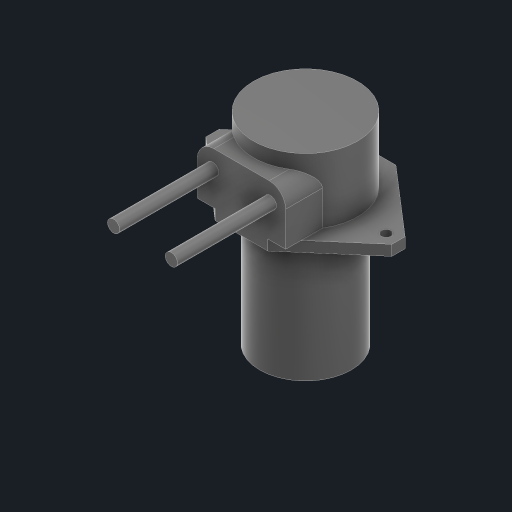
# Autodesk Inventor part: Peristaltic Pump
Saved by Autodesk Inventor 2023.1 (Build 271208000, 208)
## iProperties
Created: 2022-11-29
Part Number: Peristaltic Pump
Material: Acetal Resin, Black
Document SubType Name: Modeling
Designer: Jarrett
Density: 1.425 g/cm^3
Appearance: Smooth - Black
Author: Jarrett
Autodesk Inventor part; units mm, degrees
ref_plane "YZ Plane" through (0, 0, 0) normal (1, 0, 0) x (0, 1, 0)
ref_plane "XZ Plane" through (0, 0, 0) normal (0, 1, 0) x (-1, 0, 0)
ref_plane "XY Plane" through (0, 0, 0) normal (0, 0, 1) x (1, 0, 0)
sketch "Sketch1" plane through (0, 0, 0) normal (0, 1, 0) x (-1, 0, 0)
  line L0 (0, -19.39) -> (-8, -19.39)
  line L1 (-28.18, -2) -> (-28.18, 2)
  line L2 (-28.18, 2) -> (-8, 19.39)
  line L3 (-8, 19.39) -> (0, 19.39)
  circle A0 centre (-24.43, 0) radius 1.5
  circle A1 centre (0, 0) radius 15.75
  line L4 (0, -27.146) -> (0, 27.146) projected
  line L5 (-8, -19.39) -> (-28.18, -2)
  line L6 (39.452, 0) -> (-39.452, 0) projected
  line L7 (-13.385, 8.3009) -> (-13.385, 19.39)
  line L8 (-13.385, 19.39) -> (-8, 19.39)
  line L9 (0, -19.39) -> (8, -19.39)
  line L10 (28.18, -2) -> (28.18, 2)
  line L11 (28.18, 2) -> (8, 19.39)
  line L12 (8, 19.39) -> (0, 19.39)
  circle A2 centre (24.43, 0) radius 1.5
  line L13 (8, -19.39) -> (28.18, -2)
  line L14 (13.385, 8.3009) -> (13.385, 19.39)
  line L15 (13.385, 19.39) -> (8, 19.39)
  circle A3 centre (0, 0) radius 13.86
  point P0 (-28.18, 0)
  dimension "d4" = 31.5
  dimension "d0" = 56.36
  dimension "d1" = 38.78
  dimension "d2" = 4
  dimension "d3" = 16
  dimension "d5" = 26.77
  dimension "d6" = 3
  dimension "d7" = 3.75
  dimension "d8" = 27.72
  constraints: 28 end point, 7 symmetric about line, 3 centre point, 2 coincident, 2 perpendicular, 2 point on line, 1 equal length, 1 horizontal, 1 midpoint, 1 parallel, 1 vertical, 5 other
  measures "d0" diameter of L1 L4
  measures "d1" distance between parallel lines of L3 L0
  measures "d2" distance of L1.start L1.end
  measures "d3" diameter of L0.end L4
  measures "d5" diameter of L7 L4
  measures "d6" diameter of A0
  measures "d7" distance from line of A0.centre L1
  measures "d8" diameter of A3
extrude "Extrusion1" add sketch "Sketch1" along normal blind 3.16 contours L0 L5 L1 L6 A0 A1 L4 | L4 A1 L6 A2 L10 L13 L9 | L4 A3 L6 A1 | A1 L6 A3 L4 | L6 A0 L1 L2 L7 A1 | A1 L4 A3 L6 | L6 A3 L4 A1 | A1 L14 L11 L10 L6 A2 | A3 L6 L4 | L4 L6 A3 | L7 L2 L3 L4 A1 | A3 L4 L6 | A1 L4 L12 L11 L14 | L6 L4 A3
extrude "Extrusion2" add sketch "Sketch1" along normal blind 23 contours L4 A3 L6 A1 | A1 L6 A3 L4 | A1 L4 A3 L6 | L6 A3 L4 A1 | A3 L6 L4 | L4 L6 A3 | A3 L4 L6 | L6 L4 A3
extrude "Extrusion3" add sketch "Sketch1" along normal blind 15.5 from surface at 3.16 contours L7 L2 L3 L4 A1 | A1 L4 L12 L11 L14 | L7 L8 L2 | L11 L15 L14
extrude "Extrusion4" add sketch "Sketch1" against normal blind 38 contours A3 L6 L4 | L4 L6 A3 | A3 L4 L6 | L6 L4 A3
sketch "Sketch2" plane through (-8, 0, 19.39) normal (0, 0, 1) x (1, 0, 0)
  circle A0 centre (-0.75, 13.16) radius 1.85
  circle A1 centre (16.75, 13.16) radius 1.85
  line L0 (-0.75, 13.16) -> (16.75, 13.16) construction
  line L1 (21.385, 18.66) -> (-5.385, 18.66) projected
  line L2 (8, 13.16) -> (8, 18.66) construction
  line L3 (21.385, 18.66) -> (-5.385, 18.66) projected
  point P0 (8, 0)
  dimension "d17" = 5.5
  dimension "d18" = 17.5
  dimension "d19" = 3.7
  dimension "d20" = 3.7
  constraints: 4 end point, 2 centre point, 2 midpoint, 1 horizontal, 1 perpendicular
  measures "d17" distance between parallel lines of L1 L0
  measures "d18" distance of L0.start L0.end
  measures "d19" diameter of A0
  measures "d20" diameter of A1
extrude "Extrusion5" add sketch "Sketch2" along normal blind 30
fillet "Fillet1" radius 5 2 edges at (-13.385, 18.66, 13.8454) (13.385, 18.66, 13.8454)
body "Solid1"
